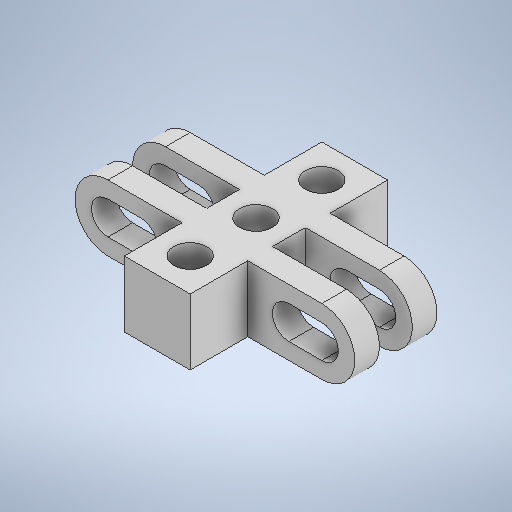
# Autodesk Inventor part: 08
Saved by Autodesk Inventor 2025.1 (Build 291241000, 241)
## iProperties
Created: 2024-09-13
Part Number: 08
Material: Generisch
Document SubType Name: Modeling
Designer: ffogue
Density: 1 g/cm^3
Appearance: Vorgabe
Author: ffogue
Autodesk Inventor part; units mm, degrees
ref_plane "YZ Plane" through (0, 0, 0) normal (1, 0, 0) x (0, 1, 0)
ref_plane "XY Plane" through (0, 0, 0) normal (0, 0, 1) x (1, 0, 0)
sketch "Sketch1" plane through (0, 0, 0) normal (0, 0, 1) x (1, 0, 0)
  line L0 (-4, -12) -> (4, -12)
  line L1 (4, -12) -> (4, 12)
  line L2 (4, 12) -> (-4, 12)
  line L3 (-4, 12) -> (-4, -12)
  line L4 (-4, -12) -> (4, 12) construction
  line L5 (4, -12) -> (-4, 12) construction
  point P0 (0, 0)
  dimension "d0" = 8
  dimension "d1" = 24
  constraints: 12 end point, 2 midpoint, 2 parallel, 1 horizontal, 1 perpendicular
  measures "d0" distance of L1.end L2.end
  measures "d1" distance of L2.end L0.start
extrude "Extrusion1" add sketch "Sketch1" along normal mid plane 8
ref_plane "Work Plane1" through (0, -2, 0) normal (0, 1, 0) x (-1, 0, 0)
sketch "Sketch3" plane through (0, -2, 0) normal (0, 1, 0) x (-1, 0, 0)
  line L0 (4, -4) -> (4, 4) projected
  line L1 (4, 4) -> (13, 4)
  arc A0 (13, -4) -> (13, 4) centre (13, 0) ccw
  line L2 (13, -4) -> (4, -4)
  line L3 (4, 4) -> (4, -4)
  line L4 (9, 0) -> (13, 0) construction
  line L5 (9, -2) -> (13, -2)
  line L6 (13, 2) -> (9, 2)
  arc A1 (9, 2) -> (9, -2) centre (9, 0) ccw
  arc A2 (13, -2) -> (13, 2) centre (13, 0) ccw
  point P0 (0, 0)
  point P1 (11, 0)
  dimension "d8" = 4
  dimension "d9" = 9
  dimension "d10" = 4
  dimension "d11" = 2
  constraints: 14 end point, 6 point on circle, 6 tangent, 3 centre point, 3 equal length, 2 horizontal, 1 coincident, 1 horizontal alignment, 1 midpoint, 1 point on line, 1 vertical alignment
  measures "d8" radius of A0
  measures "d9" distance of L4.start point (0, 0)
  measures "d10" distance of L4.start L4.end
  measures "d11" radius of A2
extrude "Extrusion2" add sketch "Sketch3" against normal blind 3
mirror "Mirror1" about plane through (0, 0, 0) normal (0, 1, 0) of "Extrusion2"
mirror "Mirror2" about plane through (0, 0, 0) normal (1, 0, 0) of "Extrusion2", "Mirror1"
sketch "Sketch4" plane through (0, 0, 4) normal (0, 0, 1) x (1, 0, 0)
  point P0 (0, 0)
  point P1 (0, -8)
  point P2 (0, 0)
  point P3 (0, 8)
  dimension "d14" = 8
  dimension "d15" = 8
  constraints: 2 vertical alignment, 1 coincident
  measures "d14" distance of point (0, 0) point (0, 8)
  measures "d15" distance of point (0, -8) point (0, 0)
hole "Hole1" at (0, -8, 4) at (0, 0, 4) at (0, 8, 4) direction (0, 0, -1) diameter 4 depth 8
sketch "Sketch5" plane through (4, -5, -4) normal (0, -1, 0) x (1, 0, 0)
  arc A0 (9, 2) -> (9, 6) centre (9, 4) ccw projected
  circle A1 centre (-14, 4) radius 2
  arc A2 (-13, 2) -> (-13, 6) centre (-13, 4) ccw projected
  arc A3 (-17, 6) -> (-17, 2) centre (-17, 4) ccw projected
  circle A4 centre (-14, 4) radius 2
  point P0 (-4, 4)
  point P1 (11, 4)
  point P2 (-11, 4)
  point P3 (-19, 4)
  dimension "d25" = 4
  dimension "d26" = 5
  constraints: 3 point on circle, 2 centre point, 1 coincident, 1 concentric, 1 horizontal alignment
  measures "d25" diameter of A1
  measures "d26" distance of point (-19, 4) A1.centre
sketch "Sketch6" plane through (-13, 5, -4) normal (0, 1, 0) x (1, 0, 0)
  arc A0 (0, -2) -> (0, -6) centre (0, -4) ccw projected
  circle A1 centre (23, -4) radius 2
  arc A2 (26, -6) -> (26, -2) centre (26, -4) ccw projected
  arc A3 (22, -2) -> (22, -6) centre (22, -4) ccw projected
  point P0 (13, -4)
  point P1 (-2, -4)
  point P2 (28, -4)
  point P3 (20, -4)
  point P4 (28, -4)
  dimension "d28" = 4
  dimension "d31" = 5
  constraints: 4 point on circle, 1 centre point, 1 horizontal alignment
  measures "d28" diameter of A1
  measures "d31" distance of point (28, -4) A1.centre
equation "\"d15\" = d14"
body "Solid1"
